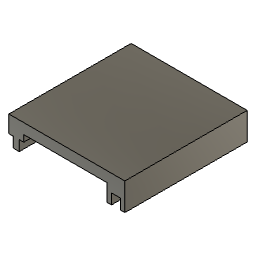
Flex_holder_2 (Autodesk Fusion 360 design; units mm, degrees)
Autodesk Fusion 360 part; units mm, degrees
sketch "Sketch1" plane through (0, 22, 0) normal (0, 1, 0) x (-1, 0, 0)
  line L0 (11.5698, 0.25) -> (15.3, 0.25)
  line L1 (15.3, 0.25) -> (15.3, -0.5)
  line L2 (15.3, -0.5) -> (15.6004, -0.5)
  line L3 (15.6004, -0.5) -> (15.6004, -1.2)
  line L4 (15.6004, -1.2) -> (16.0004, -1.2)
  line L5 (16.0004, -1.2) -> (16.0004, -0.5)
  line L6 (16.0004, -0.5) -> (16.3, -0.5)
  line L7 (16.3, -0.5) -> (16.3, 1.05)
  line L8 (16.3, 1.05) -> (5, 1.05)
  line L9 (11.5698, -1.2) -> (11.5698, 0.25)
  line L10 (11.5698, -0.6208) -> (11.2698, -0.6208) construction
  line L11 (11.2698, -0.5) -> (11.2698, -1.2)
  line L12 (11.2698, -0.5) -> (10.5698, -0.5)
  line L13 (10.5698, -0.5) -> (10.5698, -1.2)
  line L14 (10.5698, -0.678) -> (10.2698, -0.678) construction
  line L15 (10.2698, 1.05) -> (10.2698, -1.2)
  line L16 (10.2698, 1.05) -> (16.3, 1.05)
  line L17 (16.3, -0.5) -> (16.0004, -0.5)
  line L18 (16.0004, -1.2) -> (15.6004, -1.2)
  line L19 (15.6004, -0.5) -> (15.3, -0.5)
  line L20 (15.3, 0.25) -> (11.5698, 0.25)
  line L21 (11.5698, -1.2) -> (11.2698, -1.2)
  line L22 (11.5698, -1.2) -> (11.2698, -1.2)
  line L23 (11.2698, -0.5) -> (10.5698, -0.5)
  line L24 (10.5698, -1.2) -> (10.2698, -1.2)
  line L25 (10.2698, 1.05) -> (16.3, 1.05)
  line L26 (16.3, -0.5) -> (16.0004, -0.5)
  line L27 (16.0004, -1.2) -> (15.6004, -1.2)
  line L28 (15.6004, -0.5) -> (15.3, -0.5)
  line L29 (15.3, 0.25) -> (11.5698, 0.25)
  dimension "d14" = 0.3
  dimension "d15" = 0.7
  dimension "d16" = 0.3
  constraint coincident L9 L10.start
  constraint perpendicular L9 L10
  constraint perpendicular L11 L12
  constraint coincident L13 L14.start
  constraint perpendicular L13 L14
  constraint coincident L8 L15.start
  constraint coincident L7.end L8.start
  constraint coincident L6.end L7.start
  constraint coincident L5.end L6.start
  constraint coincident L4.end L5.start
  constraint coincident L3.end L4.start
  constraint coincident L2.end L3.start
  constraint coincident L1.end L2.start
  constraint coincident L0.end L1.start
  constraint coincident L0.start L9.end
  constraint coincident L9.start L21.start
  constraint perpendicular L11 L21
  constraint perpendicular L13 L23
  constraint perpendicular L15 L24
  constraint perpendicular L7 L25
  measures "d14" distance of L10.start L10.end
  measures "d15" distance of L11.start L12.end
  measures "d16" distance of L14.start L14.end
extrude "Extrude1" add sketch "Sketch1" along normal blind 8.2 makes body 1
copy_body "Body->Comp1" bodies 1 removing the originals makes body 2 in component "Component"
move_face "OffsetFaces1" offset 0.3 1 faces at (-12.8132, 24.7333, 0.25) on bodies 2 in component "Component"
move_face "OffsetFaces2" offset -0.4 1 faces at (-12.2798, 27.4667, 1.05) on bodies 2 in component "Component"
move_face "OffsetFaces3" offset 3.3 1 faces at (-10.2698, 24.7333, 0.0333) on bodies 2 in component "Component"
move_face "OffsetFaces4" offset -3.3 1 faces at (-10.5698, 24.7333, -0.7333) on bodies 2 in component "Component"
move_face "OffsetFaces5" offset 3.3 1 faces at (-11.2698, 24.7333, -0.7333) on bodies 2 in component "Component"
move_face "OffsetFaces6" offset -3.3 1 faces at (-11.5698, 27.4667, -0.8167) on bodies 2 in component "Component"
move_face "OffsetFaces7" offset -4.2 1 faces at (-10.5132, 22, 0.4167) on bodies 2 in component "Component"
move_face "OffsetFaces8" offset -0.1 1 faces at (-8.2698, 28.8667, -0.4333) on bodies 2 in component "Component"
move_face "OffsetFaces9" offset 0.1 1 faces at (-7.9698, 27.5333, -0.7333) on bodies 2 in component "Component"
move_face "OffsetFaces10" offset 4.255 1 faces at (-10.4798, 26.2, 0.4167) on bodies 2 in component "Component"
move_face "OffsetFaces11" offset 0.3 1 faces at (-6.9698, 24.6967, 0.0333) on bodies 2 in component "Component"
move_face "OffsetFaces12" offset 0.3 1 faces at (-7.8698, 24.6967, -0.7333) on bodies 2 in component "Component"
move_face "OffsetFaces13" offset -0.3 1 faces at (-7.2698, 24.6967, -0.7333) on bodies 2 in component "Component"
move_face "OffsetFaces14" offset -0.3 1 faces at (-8.1698, 24.6967, -0.8167) on bodies 2 in component "Component"
move_face "OffsetFaces15" offset 1.8 2 faces at (-15.3, 24.6967, -0.2) (-15.6004, 24.6967, -0.7333) on bodies 2 in component "Component"
move_face "OffsetFaces16" offset -1.8 2 faces at (-16.0004, 24.6967, -0.9667) (-16.3, 24.6967, -0.1167) on bodies 2 in component "Component"
component "Component" placed x (1, 0, 0) y (0, 1, 0) z (0, 0, 1) at (0, 0, 0)
